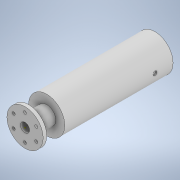
# Autodesk Inventor part: again
Saved by Autodesk Inventor 2022 (Build 260153000, 153)
## iProperties
Created: 2022-03-10
Part Number: again
Material: Generic
Document SubType Name: Modeling
Designer: karee
Density: 1 g/cm^3
Appearance: Default
Author: karee
Autodesk Inventor part; units mm, degrees
ref_plane "XZ Plane" through (0, 0, 0) normal (0, 1, 0) x (-1, 0, 0)
ref_plane "XY Plane" through (0, 0, 0) normal (0, 0, 1) x (1, 0, 0)
sketch "Sketch1" plane through (0, 0, 0) normal (0, 0, 1) x (1, 0, 0)
  circle A0 centre (0, 0) radius 50
  dimension "d0" = 100
  constraints: 1 centre point, 1 coincident
  measures "d0" diameter of A0
extrude "Extrusion1" add sketch "Sketch1" along normal blind 300
sketch "Sketch2" plane through (0, 0, 300) normal (0, 0, 1) x (1, 0, 0)
  circle A0 centre (0, 0) radius 50 projected
  circle A1 centre (0, 0) radius 46
  dimension "d3" = 92
  constraints: 1 centre point, 1 coincident
  measures "d3" diameter of A1
extrude "Extrusion2" cut sketch "Sketch2" against normal blind 296 contours A1
sketch "Sketch3" plane through (0, 0, 300) normal (0, 0, 1) x (1, 0, 0)
  circle A0 centre (0, 0) radius 46
  constraints: 1 centre point, 1 coincident
extrude "Extrusion3" add sketch "Sketch3" against normal blind 4
sketch "Sketch4" plane through (0, 0, 300) normal (0, 0, 1) x (1, 0, 0)
  circle A0 centre (0, 0) radius 25
  dimension "d8" = 50
  constraints: 1 centre point, 1 coincident
  measures "d8" diameter of A0
extrude "Extrusion4" add sketch "Sketch4" along normal blind 50
sketch "Sketch5" plane through (0, 0, 350) normal (0, 0, 1) x (1, 0, 0)
  circle A0 centre (0, 0) radius 12.5
  dimension "d11" = 25
  constraints: 1 centre point, 1 coincident
  measures "d11" diameter of A0
extrude "Extrusion5" cut sketch "Sketch5" against normal blind 100
sketch "Sketch6" plane through (0, 0, 350) normal (0, 0, 1) x (1, 0, 0)
  circle A0 centre (0, 0) radius 50
  constraints: 1 centre point, 1 coincident
extrude "Extrusion6" add sketch "Sketch6" along normal blind 10
sketch "Sketch7" plane through (0, 0, 360) normal (0, 0, 1) x (1, 0, 0)
  circle A0 centre (0, 0) radius 12.5 projected
  circle A1 centre (0, 0) radius 12.5
  constraints: 1 centre point, 1 coincident
extrude "Extrusion7" cut sketch "Sketch7" against normal blind 300
sketch "Sketch8" plane through (0, 0, 360) normal (0, 0, 1) x (1, 0, 0)
  line L0 (0, 0) -> (0, -36)
  line L1 (0, 0) -> (0, 36)
  line L2 (0, 0) -> (36, 0)
  line L3 (0, 0) -> (-36, 0)
  circle A0 centre (0, 0) radius 12.5 projected
  line L4 (0, 0) -> (0, 36)
  circle A1 centre (0, 36) radius 4
  dimension "d31" = 8
  constraints: 10 end point, 3 vertical, 2 horizontal, 1 centre point, 1 coincident
  measures "d31" diameter of A1
ref_plane "Work Plane1" through (50, 0, 0) normal (1, 0, 0) x (0, 1, 0)
extrude "Extrusion9" cut sketch "Sketch8" along normal mid plane 25 contours A1
sketch "Sketch11" plane through (0, 0, 360) normal (0, 0, 1) x (1, 0, 0)
  point P0 (0, 0)
pattern_circular "Circular Pattern1" count 6 over 360 about axis through (0, 0, 350) along (0, 0, -1) of "Extrusion9"
sketch "Sketch12" plane through (50, 0, 0) normal (1, 0, 0) x (0, 1, 0)
  line L0 (0, 0) -> (0, 50)
  circle A0 centre (0, 50) radius 5.5
  dimension "d37" = 50
  dimension "d39" = 11
  constraints: 2 end point, 1 centre point, 1 coincident
  measures "d37" distance of L0.start L0.end
  measures "d39" diameter of A0
extrude "Extrusion10" cut sketch "Sketch12" against normal blind 50
body "Solid1"
